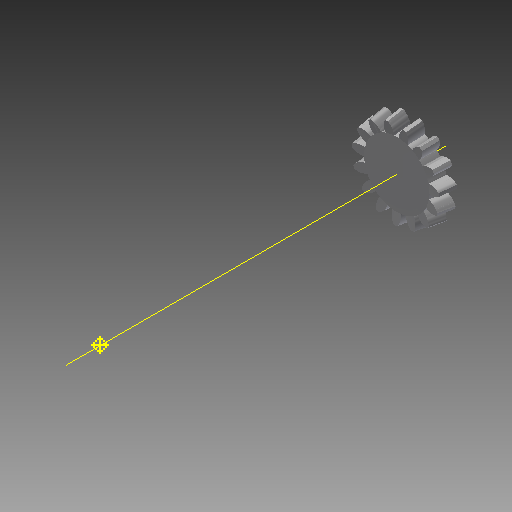
# Autodesk Inventor part: Bevel Gear2
Saved by Autodesk Inventor 2017 (Build 210142000, 142)
## iProperties
Created: 2017-01-10
Part Number: Bevel Gear2
Material: Steel, Mild
Document SubType Name: Modeling
Designer: David Kopala
Categories: <?xml version="1.0" encoding="UTF-16"?> <MemberInstance><Categories><FamilyTemplate><FamilyTemplateParameter ValueType="xs:double" Id="1" ObjectReferenceKey="da_z" ObjectType="kUserParameterObject"/><FamilyTemplateParameter ValueType="xs:double" Id="2" ObjectReferenceKey="da_b" ObjectType="kUserParameterObject"/><FamilyTemplateParameter ValueType="xs:double" Id="3" ObjectReferenceKey="da_beta" ObjectType="kUserParameterObject"/><FamilyTemplateParameter ValueType="xs:double" Id="4" ObjectReferenceKey="da_dae" ObjectType="kUserParameterObject"/><FamilyTemplateParameter ValueType="xs:double" Id="5" ObjectReferenceKey="da_ve" ObjectType="kUserParameterObject"/><FamilyTemplateParameter ValueType="xs:double" Id="6" ObjectReferenceKey="da_omega" ObjectType="kUserParameterObject"/><FamilyTemplateParameter ValueType="xs:string" Id="7" ObjectReferenceKey="EAIAABAAAAAAHwAAAAAAAIAAAAAAAAAA" ObjectType="83914240" SubObjectId="SurfaceGeometry"/></FamilyTemplate><ParamToTemplateMap><ParamToTemplate CategoryParameter="//CategoryParameter[@InternalName='046C89C9-8512-4d59-83FE-43B91F4F132A']" TemplateParameter="1"/><ParamToTemplate CategoryParameter="//CategoryParameter[@InternalName='2552DF32-E462-4b46-AEBF-C6C7768E72AC']" TemplateParameter="2"/><ParamToTemplate CategoryParameter="//CategoryParameter[@InternalName='C9EE641D-15FC-4fae-A226-E94C4372FDD7']" TemplateParameter="3"/><ParamToTemplate><ParamToTemplate CategoryParameter="//CategoryParameter[@InternalName='00B6519A-459B-49c7-AD84-2E56D39A5744']" ConstantValue="-0.000000"/></ParamToTemplate><ParamToTemplate><ParamToTemplate CategoryParameter="//CategoryParameter[@InternalName='04B31F0E-C7A6-4894-AA32-9629BEFACF47']" ConstantValue="1.000000"/></ParamToTemplate><ParamToTemplate><ParamToTemplate CategoryParameter="//CategoryParameter[@InternalName='43CBEC2E-7847-49e7-A936-2F7889FCB2D9']" ConstantValue="0.200000"/></ParamToTemplate><ParamToTemplate><ParamToTemplate CategoryParameter="//CategoryParameter[@InternalName='B1EFC894-105D-4ebd-86BF-FA20ED196853']" ConstantValue="0.300000"/></ParamToTemplate><ParamToTemplate><ParamToTemplate CategoryParameter="//CategoryParameter[@InternalName='51175063-3D10-4879-93E8-6246FE8B403D']" ConstantValue="2061532430.657340"/></ParamToTemplate><ParamToTemplate><ParamToTemplate CategoryParameter="//CategoryParameter[@InternalName='A3A52E27-4454-46a9-B0BD-C932399B70AF']" ConstantValue="0.300000"/></ParamToTemplate><ParamToTemplate CategoryParameter="//CategoryParameter[@InternalName='2A200944-5A8C-41ca-B96E-8520D2E510F1']" TemplateParameter="4"/><ParamToTemplate><ParamToTemplate CategoryParameter="//CategoryParameter[@InternalName='1A637F62-92C8-44bc-B81F-10802510B579']" ConstantValue="4.072666"/></ParamToTemplate><ParamToTemplate CategoryParameter="//CategoryParameter[@InternalName='B52DD4BE-6863-48fb-BF58-89EF6F9EC65C']" TemplateParameter="5"/><ParamToTemplate><ParamToTemplate CategoryParameter="//CategoryParameter[@InternalName='3956BFF2-84D2-457d-93C2-9B0613DEBA67']" ConstantValue="13.819415"/></ParamToTemplate><ParamToTemplate CategoryParameter="//CategoryParameter[@InternalName='739CFA02-461B-4bf8-8049-181FCAD8B28F']" TemplateParameter="6"/><ParamToTemplate><ParamToTemplate CategoryParameter="//CategoryParameter[@InternalName='A27E999F-E2CE-4481-8A2A-EBF499C4C3C5']" ConstantValue="-0.000000"/></ParamToTemplate><ParamToTemplate><ParamToTemplate CategoryParameter="//CategoryParameter[@InternalName='9E1B4470-B2D3-4ff1-B813-535BB4CDF51A']" ConstantValue="3523220.976809"/></ParamToTemplate><ParamToTemplate><ParamToTemplate CategoryParameter="//CategoryParameter[@InternalName='F8452263-BFF6-458c-9FB1-07C4B99E95CD']" ConstantValue="11397033.805607"/></ParamToTemplate><ParamToTemplate><ParamToTemplate CategoryParameter="//CategoryParameter[@InternalName='3E3BB259-FD49-497f-8171-6EBC954A3479']" ConstantValue="2.000000"/></ParamToTemplate><ParamToTemplate CategoryParameter="//CategoryParameter[@InternalName='27C3BAF2-7550-4e4b-AE2C-0DB134B7D9B7']" TemplateParameter="7"/></ParamToTemplateMap><Category DisplayName="Gear" InternalName="DC85795E-93AB-48d5-8EEE-5A27447B64BD" Mnemonic="Gear"><CategoryParameter DisplayName="z" InternalName="046C89C9-8512-4d59-83FE-43B91F4F132A" Mnemonic="z"/><CategoryParameter DisplayName="b" InternalName="2552DF32-E462-4b46-AEBF-C6C7768E72AC" Mnemonic="b"/><CategoryParameter DisplayName="||b|" InternalName="C9EE641D-15FC-4fae-A226-E94C4372FDD7" Mnemonic="beta"/><CategoryParameter DisplayName="x" InternalName="00B6519A-459B-49c7-AD84-2E56D39A5744" Mnemonic="x"/><CategoryParameter DisplayName="a*" InternalName="04B31F0E-C7A6-4894-AA32-9629BEFACF47" Mnemonic="a"/><CategoryParameter DisplayName="c*" InternalName="43CBEC2E-7847-49e7-A936-2F7889FCB2D9" Mnemonic="c"/><CategoryParameter DisplayName="r|.f|*" InternalName="B1EFC894-105D-4ebd-86BF-FA20ED196853" Mnemonic="rf"/><CategoryParameter DisplayName="E" InternalName="51175063-3D10-4879-93E8-6246FE8B403D" Mnemonic="E"/><CategoryParameter DisplayName="||m|" InternalName="A3A52E27-4454-46a9-B0BD-C932399B70AF" Mnemonic="mi"/><Category DisplayName="BevelGear" InternalName="0C98F69A-0C2B-4791-B2FE-7691BB227E77" Mnemonic="BevelGear"><CategoryParameter DisplayName="d|.ae|" InternalName="2A200944-5A8C-41ca-B96E-8520D2E510F1" Mnemonic="dae"/><CategoryParameter DisplayName="d|.ai|" InternalName="1A637F62-92C8-44bc-B81F-10802510B579" Mnemonic="dai"/><CategoryParameter DisplayName="A|.e|" InternalName="B52DD4BE-6863-48fb-BF58-89EF6F9EC65C" Mnemonic="ve"/><CategoryParameter DisplayName="A|.i|" InternalName="3956BFF2-84D2-457d-93C2-9B0613DEBA67" Mnemonic="vi"/><CategoryParameter DisplayName="||S|" InternalName="739CFA02-461B-4bf8-8049-181FCAD8B28F" Mnemonic="omega"/><CategoryParameter DisplayName="x|.t|" InternalName="A27E999F-E2CE-4481-8A2A-EBF499C4C3C5" Mnemonic="xt"/><CategoryParameter DisplayName="||s||.Flim|" InternalName="9E1B4470-B2D3-4ff1-B813-535BB4CDF51A" Mnemonic="sFlim"/><CategoryParameter DisplayName="||s||.Hlim|" InternalName="F8452263-BFF6-458c-9FB1-07C4B99E95CD" Mnemonic="sHlim"/><CategoryParameter DisplayName="type" InternalName="3E3BB259-FD49-497f-8171-6EBC954A3479" Mnemonic="type"/><CategoryParameter DisplayName="PitchDiameter" InternalName="27C3BAF2-7550-4e4b-AE2C-0DB134B7D9B7" Mnemonic="IDS_PITCHDIAM"/></Category></Category></Categories></MemberInstance>
Mass: 60.9118 g
Surface Area: 34.3074 cm^2
Volume: 7.7496 cm^3
Density: 7.86 g/cm^3
Appearance: Steel
CustomPartVersion: 1
Author: David Kopala
Autodesk Inventor part; units mm, degrees
ref_plane "XZ Plane" through (0, 0, 0) normal (0, 1, 0) x (-1, 0, 0)
ref_plane "Mesh Plane2" through (0, 0, 0) normal (0.9781476, 0.2079117, 0) x (0, 0, 1)
sketch "Teeth Body Sketch" plane through (0, 0, 0) normal (1, 0, 0) x (0, 1, 0)
  line L0 (0, 0) -> (16.0276, -146.4442) construction
  line L1 (16.0276, -146.4442) -> (21.4743, -145.7338)
  line L2 (21.4743, -145.7338) -> (0, 0) construction
  line L3 (19.05, -146.05) -> (0, 0) construction
  line L4 (15.1984, -138.8678) -> (20.3633, -138.1941)
  line L5 (16.0276, -146.4442) -> (15.1984, -138.8678)
  line L6 (21.4743, -145.7338) -> (20.3633, -138.1941)
  line L7 (0, -177.2531) -> (0, 29.5422) projected
  line L8 (0, -146.05) -> (21.4743, -146.05) construction
  dimension "d0" = 38.1
  dimension "d1" = 32.0552
  dimension "d2" = 42.9486
  dimension "d3" = 7.62
  dimension "d4" = 145.7338
  constraints: 16 end point, 4 point on line, 3 perpendicular, 2 collinear, 1 horizontal alignment, 1 vertical alignment
  measures "d0" diameter of L3.start L7
  measures "d1" diameter of L0.end L7
  measures "d2" diameter of L1.end L7
  measures "d3" distance between parallel lines of L1 L4
  measures "d4" vertical distance of L1.end L0.start
revolve "Teeth Body" add sketch "Teeth Body Sketch" angle 360 about axis through (0, 0, 0) along (0, 0, 1)
ref_plane "Tooth Plane" through (0, 19.05, -146.05) normal (0, -0.1293392, 0.9916004) x (1, 0, 0)
sketch "Start Sketch" plane through (0, 19.05, -146.05) normal (0, -0.1293392, 0.9916004) x (1, 0, 0)
  line L0 (0, -23.8689) -> (0, 8.7531) projected
  arc A0 (-1.2145, -3.7071) -> (-5.7859, 3.363) centre (-8.4705, -3.3857) ccw
  arc A1 (5.7859, 3.363) -> (1.2145, -3.7071) centre (8.4705, -3.3857) ccw
  line L1 (-1.2145, -3.7071) -> (1.2145, -3.7071)
  arc A2 (5.7859, 3.363) -> (-5.7859, 3.363) centre (0, -19.2114) ccw
  dimension "d7" = 7.2631
  dimension "d8" = 8.4705
  dimension "d9" = 15.8257
  dimension "d57" = 23.3041
  dimension "d58" = 15.5042
  constraints: 6 point on circle, 3 centre point, 3 symmetric about line, 2 end point, 1 coincident, 1 perpendicular, 1 other
  measures "d7" radius of A0
  measures "d8" horizontal distance of point (0, -19.211) A0.centre
  measures "d9" vertical distance of point (0, -19.211) A0.centre
  measures "d57" radius of A2
  measures "d58" distance from line of A2.centre L1
sketch "End Sketch" plane through (0, 18.0289, -138.2217) normal (0, -0.1293392, 0.9916004) x (1, 0, 0)
  line L0 (0, -22.605) -> (0, 8.3159) projected
  arc A0 (-1.1506, -3.4929) -> (-5.4815, 3.2054) centre (-8.025, -3.1884) ccw
  arc A1 (5.4815, 3.2054) -> (1.1506, -3.4929) centre (8.025, -3.1884) ccw
  line L1 (-1.1506, -3.4929) -> (1.1506, -3.4929)
  arc A2 (5.4815, 3.2054) -> (-5.4815, 3.2054) centre (0, -18.1816) ccw
  dimension "d12" = 6.8811
  dimension "d15" = 8.025
  dimension "d16" = 14.9932
  dimension "d59" = 22.0783
  dimension "d60" = 14.6887
  constraints: 6 point on circle, 3 centre point, 3 symmetric about line, 2 end point, 1 coincident, 1 other
  measures "d12" radius of A0
  measures "d15" horizontal distance of A0.centre point (0, -18.182)
  measures "d16" vertical distance of A0.centre point (0, -18.182)
  measures "d59" radius of A2
  measures "d60" distance from line of A2.centre L1
loft "Loft" cut profiles "Start Sketch", "End Sketch"
pattern_circular "Circular Pattern" count 15 over 360 about axis through (0, 0, 0) along (0, 0, 1) of "Loft"
ref_plane "End Plane" through (0, 18.0289, -138.2217) normal (0, -0.1293392, 0.9916004) x (1, 0, 0)
sketch3d "3D Sketch Right"
ref_plane "End Plane Right" through (-2.8108, 17.8085, -138.2217) normal (0.0201644, -0.1277577, 0.9916004) x (0.9877723, 0.1559034, 0)
sketch "End Sketch Right" plane through (-2.8108, 17.8085, -138.2217) normal (0.0201644, -0.1277577, 0.9916004) x (0.9877723, 0.1559034, 0)
  arc A0 (-1.1506, -3.4929) -> (-5.4815, 3.2054) centre (-8.025, -3.1884) ccw
  line L0 (0, -26.0375) -> (0, 11.7483) projected
  arc A1 (5.4815, 3.2054) -> (1.1506, -3.4929) centre (8.025, -3.1884) ccw
  line L1 (-1.1506, -3.4929) -> (1.1506, -3.4929)
  arc A2 (5.4815, 3.2054) -> (-5.4815, 3.2054) centre (0, -18.1816) ccw
  dimension "d70" = 8.025
  dimension "d71" = 14.9932
  dimension "d72" = 6.8811
  dimension "d73" = 14.6887
  dimension "d74" = 22.0783
  constraints: 6 point on circle, 3 centre point, 3 symmetric about line, 2 end point, 1 coincident, 1 perpendicular, 1 other
  measures "d70" horizontal distance of A2.centre A0.centre
  measures "d71" vertical distance of point (0, -18.182) A0.centre
  measures "d72" radius of A0
  measures "d73" distance from line of point (0, -18.182) L1
  measures "d74" radius of A2
feature "Loft Right" [suppressed]
pattern_circular "Circular Pattern Right" [suppressed]
sketch3d "3D Sketch Left"
ref_plane "End Plane Left" through (2.7996, 17.8085, -138.2177) normal (-0.0200846, -0.1277615, 0.9916015) x (0.9878679, -0.1552965, 0)
sketch "End Sketch Left" plane through (2.7996, 17.8085, -138.2177) normal (-0.0200846, -0.1277615, 0.9916015) x (0.9878679, -0.1552965, 0)
  line L0 (0, -55.1646) -> (0, 20.9754) projected
  arc A0 (-1.1506, -3.4917) -> (-5.4815, 3.2066) centre (-8.025, -3.1872) ccw
  arc A1 (5.4815, 3.2066) -> (1.1506, -3.4917) centre (8.025, -3.1872) ccw
  line L1 (-1.1506, -3.4917) -> (1.1506, -3.4917)
  ellipse E0 centre (0, -17.8727) end of major axis (20.3633, -17.8727) minor radius 20.1923 projected
  arc A2 (5.4815, 3.2066) -> (-5.4815, 3.2066) centre (0, -18.1804) ccw
  dimension "d56" = 20.1923
  dimension "d30" = 6.8811
  dimension "d31" = 8.025
  dimension "d32" = 14.9932
  dimension "d61" = 22.0783
  dimension "d62" = 14.6887
  constraints: 6 point on circle, 3 centre point, 3 symmetric about line, 2 end point, 1 coincident, 2 other
  measures "d30" radius of A0
  measures "d31" horizontal distance of point (0, -18.18) A0.centre
  measures "d32" vertical distance of A0.centre point (0, -18.18)
  measures "d61" radius of A2
  measures "d62" distance from line of point (0, -18.18) L1
feature "Loft Left" [suppressed]
pattern_circular "Circular Pattern Left" [suppressed]
sketch "Body Sketch" plane through (0, 0, 0) normal (1, 0, 0) x (0, 1, 0)
  line L0 (0, -149.2263) -> (0, -138.6183) projected
  line L1 (16.0276, -146.4442) -> (15.1984, -138.8678) projected
  line L2 (15.1984, -138.8678) -> (0, -138.8678)
  line L3 (16.0276, -146.4442) -> (0, -146.4442)
  constraints: 4 end point, 2 perpendicular, 2 point on line
revolve "Fix Body" add sketch "Body Sketch" angle 360 about axis through (0, 0, 0) along (0, 0, 1)
sketch "Sketch6" plane through (0, 0, 0) normal (1, 0, 0) x (0, 1, 0)
  line L0 (19.05, -146.05) -> (0, 0) projected
  line L1 (0, -176.784) -> (0, 29.464) projected
surface revolve "Pitch Diameter" sketch "Sketch6" angle 360 about axis through (0, 0, 0) along (0, 0, 1) shown no curves L0
equation "\"d0\" = da_de"
equation "\"d1\" = da_dfe"
equation "\"d2\" = da_dae"
equation "\"d3\" = da_b"
equation "\"d4\" = da_ve"
equation "\"d7\" = fd_rr"
equation "\"d8\" = fd_x"
equation "\"d9\" = fd_y"
equation "\"d57\" = 0.5 * fd_dva + 0.3 * da_he"
equation "\"d58\" = 0.5 * fd_dva - 1.12 * da_he"
equation "\"da_teethtype\" = 0"
equation "\"da_b\" = 7.62"
equation "\"da_de\" = 38.1"
equation "\"da_dae\" = 42.94864"
equation "\"da_dfe\" = 32.0552"
equation "\"da_le\" = 147.28715"
equation "\"da_omega\" = 90deg"
equation "\"da_beta\" = 0"
equation "\"da_delta\" = 7.431408deg"
equation "\"da_alpha\" = 20deg"
equation "\"da_he\" = 5.49285"
equation "\"da_ve\" = 145.73378"
equation "\"da_zv\" = 15.127061"
equation "\"fd_loft\" = da_b + 0.05 * da_he"
equation "\"fd_x\" = fd_x1 + fd_x2"
equation "\"fd_y\" = fd_y1 - fd_y2"
equation "\"fd_dd\" = fd_dva - 0.8 * da_he"
equation "\"da_dvw\" = 38.42274"
equation "\"d11\" = fd_loft"
equation "\"da_dm\" = 37.11444"
equation "\"da_x\" = 0"
equation "\"da_m\" = 2.54"
equation "\"d50\" = da_omega"
equation "\"fd_rr\" = 7.263121"
equation "\"fd_dva\" = 43.312444"
equation "\"fd_x1\" = 1.991328"
equation "\"fd_x2\" = 6.479191"
equation "\"fd_y1\" = 19.107885"
equation "\"fd_y2\" = 3.282228"
body "Solid1"
body "Srf1"
